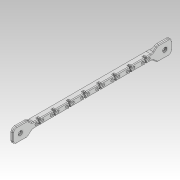
# Autodesk Inventor part: DoubleSolenoidBracket
Saved by Autodesk Inventor 2020 (Build 240168000, 168)
## iProperties
Created: 2021-09-21
Part Number: DoubleSolenoidBracket
Material: Generic
Document SubType Name: Modeling
Designer: DDeGo
Density: 1 g/cm^3
Appearance: Default
Author: DDeGo
Autodesk Inventor part; units mm, degrees
ref_plane "YZ Plane" through (0, 0, 0) normal (1, 0, 0) x (0, 1, 0)
ref_plane "XZ Plane" through (0, 0, 0) normal (0, 1, 0) x (-1, 0, 0)
sketch "Sketch1" plane through (0, 0, 0) normal (1, 0, 0) x (0, 1, 0)
  line L0 (0, 0) -> (8, 0)
  line L1 (8, 0) -> (8, -166)
  line L2 (8, -166) -> (0, -166)
  line L3 (0, -166) -> (0, 0)
  line L4 (4, 0) -> (4, -5) construction
  line L5 (4, -5) -> (4, -14) construction
  circle A0 centre (4, -5) radius 1.75
  circle A1 centre (4, -14) radius 1.75
  line L6 (2.75, -10.5) -> (2.75, -8.5) construction
  line L7 (5.25, -8.5) -> (5.25, -10.5) construction
  line L8 (8, -10.5) -> (5.25, -10.5) construction
  line L9 (2.75, -10.5) -> (0, -10.5) construction
  line L10 (0, -8.5) -> (2.75, -8.5) construction
  line L11 (5.25, -8.5) -> (8, -8.5) construction
  line L12 (5.25, -9.5) -> (2.75, -9.5) construction
  circle A2 centre (4, -35) radius 1.75
  line L13 (2.75, -31.5) -> (2.75, -29.5) construction
  line L14 (5.25, -29.5) -> (5.25, -31.5) construction
  circle A3 centre (4, -26) radius 1.75
  line L15 (4, -26) -> (4, -35) construction
  circle A4 centre (4, -56) radius 1.75
  line L16 (2.75, -52.5) -> (2.75, -50.5) construction
  line L17 (5.25, -50.5) -> (5.25, -52.5) construction
  circle A5 centre (4, -47) radius 1.75
  line L18 (4, -47) -> (4, -56) construction
  circle A6 centre (4, -77) radius 1.75
  line L19 (2.75, -73.5) -> (2.75, -71.5) construction
  line L20 (5.25, -71.5) -> (5.25, -73.5) construction
  circle A7 centre (4, -68) radius 1.75
  line L21 (4, -68) -> (4, -77) construction
  circle A8 centre (4, -98) radius 1.75
  line L22 (2.75, -94.5) -> (2.75, -92.5) construction
  line L23 (5.25, -92.5) -> (5.25, -94.5) construction
  circle A9 centre (4, -89) radius 1.75
  line L24 (4, -89) -> (4, -98) construction
  circle A10 centre (4, -119) radius 1.75
  line L25 (2.75, -115.5) -> (2.75, -113.5) construction
  line L26 (5.25, -113.5) -> (5.25, -115.5) construction
  circle A11 centre (4, -110) radius 1.75
  line L27 (4, -110) -> (4, -119) construction
  circle A12 centre (4, -140) radius 1.75
  line L28 (2.75, -136.5) -> (2.75, -134.5) construction
  line L29 (5.25, -134.5) -> (5.25, -136.5) construction
  circle A13 centre (4, -131) radius 1.75
  line L30 (4, -131) -> (4, -140) construction
  circle A14 centre (4, -161) radius 1.75
  line L31 (2.75, -157.5) -> (2.75, -155.5) construction
  line L32 (5.25, -155.5) -> (5.25, -157.5) construction
  circle A15 centre (4, -152) radius 1.75
  line L33 (4, -152) -> (4, -161) construction
  point P0 (4, -9.5)
  point P1 (5.25, -30.5)
  point P2 (2.75, -30.5)
  point P3 (4, -30.5)
  point P4 (5.25, -51.5)
  point P5 (2.75, -51.5)
  point P6 (4, -51.5)
  point P7 (5.25, -72.5)
  point P8 (2.75, -72.5)
  point P9 (4, -72.5)
  point P10 (5.25, -93.5)
  point P11 (2.75, -93.5)
  point P12 (4, -93.5)
  point P13 (5.25, -114.5)
  point P14 (2.75, -114.5)
  point P15 (4, -114.5)
  point P16 (5.25, -135.5)
  point P17 (2.75, -135.5)
  point P18 (4, -135.5)
  point P19 (5.25, -156.5)
  point P20 (2.75, -156.5)
  point P21 (4, -156.5)
  dimension "d0" = 9
  dimension "d1" = 3.5
  dimension "d2" = 5
  dimension "d3" = 2.5
  dimension "d4" = 2
  dimension "d5" = 8
  dimension "d8" = 21
  dimension "d13" = 5
  constraints: 68 end point, 16 centre point, 16 coincident, 10 perpendicular, 5 midpoint, 5 point on line, 3 parallel, 2 collinear, 1 equal radius, 1 horizontal, 1 vertical, 111 other
  measures "d0" distance of L4.end L5.end
  measures "d1" diameter of A0
  measures "d2" distance of L4.start L4.end
  measures "d3" distance between parallel lines of L6 L7
  measures "d4" distance of L7.start L7.end
  measures "d5" distance between parallel lines of L3 L1
  measures "d8" distance of A1.centre A2.centre
  measures "d13" distance from line of A14.centre L2
extrude "Extrusion1" add sketch "Sketch1" along normal blind 7
sketch "Sketch2" plane through (7, 0, 0) normal (1, 0, 0) x (0, 0, -1)
  circle A0 centre (5, 4) radius 1.75 construction
  circle A1 centre (14, 4) radius 1.75 construction
  line L0 (5, 4) -> (14, 4) construction
  line L1 (8.75, 2.75) -> (10.25, 2.75)
  line L2 (10.25, 2.75) -> (10.25, 5.25) construction
  line L3 (10.25, 5.25) -> (8.75, 5.25)
  line L4 (8.75, 5.25) -> (8.75, 2.75) construction
  line L5 (8.75, 2.75) -> (10.25, 5.25) construction
  line L6 (10.25, 2.75) -> (8.75, 5.25) construction
  line L7 (8.75, 5.25) -> (8.75, 8)
  line L8 (166, 8) -> (0, 8) construction
  line L9 (10.25, 5.25) -> (10.25, 8)
  line L10 (8.75, 8) -> (10.25, 8)
  line L11 (10.25, 2.75) -> (10.25, 0)
  line L12 (0, 0) -> (166, 0) construction
  line L13 (8.75, 2.75) -> (8.75, 0)
  line L14 (10.25, 0) -> (8.75, 0)
  point P0 (9.5, 4)
  dimension "d16" = 2.5
  dimension "d17" = 1.5
  constraints: 26 end point, 6 point on line, 3 midpoint, 3 parallel, 3 perpendicular, 2 horizontal, 1 vertical
  measures "d16" distance between parallel lines of L1 L3
  measures "d17" distance between parallel lines of L4 L2
extrude "Extrusion2" cut sketch "Sketch2" against normal blind 3.5
fillet "Fillet1" radius 1 4 edges at (5.25, 8, -8.75) (5.25, 8, -10.25) (5.25, 0, -8.75) (5.25, 0, -10.25)
fillet "Fillet1" radius 0.5 4 edges at (5.25, 2.75, -8.75) (5.25, 2.75, -10.25) (5.25, 5.25, -8.75) (5.25, 5.25, -10.25)
sketch "Sketch4" plane through (0, 0, 0) normal (-1, 0, 0) x (0, 0, 1)
  circle A0 centre (-5, 4) radius 1.75 projected
  circle A1 centre (-5, 4) radius 3
  circle A2 centre (-14, 4) radius 1.75 projected
  circle A3 centre (-14, 4) radius 3
  point P0 (0, 0)
  dimension "d25" = 6
  constraints: 2 centre point, 2 coincident, 1 equal radius
  measures "d25" diameter of A1
extrude "Extrusion4" cut sketch "Sketch4" against normal blind 3 contours A0 | A1 | A2 | A3
pattern_linear "Rectangular Pattern1" count 8 spacing 21 along (0, 0, -1) of "Extrusion4", "Extrusion2", "Fillet1"
ref_plane "Work Plane1" through (0, 0, -83) normal (0, 0, 1) x (1, 0, 0)
sketch "Sketch5" plane through (7, 0, 0) normal (1, 0, 0) x (0, 0, -1)
  line L0 (0, 0) -> (166, 0) construction
  line L1 (166, 8) -> (0, 8) construction
  line L2 (0, 0) -> (0, 8)
  line L3 (0, 8) -> (-7, 14)
  line L4 (-7, 14) -> (-27, 14)
  line L5 (-27, 14) -> (-27, -6)
  line L6 (-27, -6) -> (-7, -6)
  line L7 (-7, -6) -> (-7, 14) construction
  line L8 (0, 8) -> (0, 0) projected
  line L9 (-7, -6) -> (0, 0)
  line L10 (-7, 4) -> (-27, 4) construction
  circle A0 centre (-17, 4) radius 3
  line L11 (83, -10) -> (83, 18) projected
  dimension "d31" = 6
  dimension "d32" = 20
  dimension "d33" = 100
  dimension "d34" = 20
  constraints: 16 end point, 5 perpendicular, 3 midpoint, 1 centre point, 1 equal length
  measures "d31" diameter of A0
  measures "d32" distance of L4.end L5.end
  measures "d33" distance from line of L11 A0.centre
  measures "d34" distance of L3.end L4.end
extrude "Extrusion5" add sketch "Sketch5" against normal blind 3
mirror "Mirror1" about plane through (0, 0, -83) normal (0, 0, 1) of "Extrusion5"
fillet "Fillet2" radius 5 4 edges at (5.5, 14, 27) (5.5, -6, 27) (5.5, 14, -193) (5.5, -6, -193)
fillet "Fillet2" radius 5 8 edges at (5.5, 14, 7) (5.5, 0, 0) (5.5, 8, 0) (5.5, -6, 7) (5.5, 14, -173) (5.5, 8, -166) (5.5, 0, -166) (5.5, -6, -173)
chamfer "Chamfer1" distance 4 angle 45 2 edges at (4, 4, 0) (4, 4, -166)
fillet "Fillet3" radius 5 2 edges at (4, 4, 3.9999) (4, 4, -169.9999)
fillet "Fillet4" radius 1 152 edges at (7, 0.2929, -10.5429) (7, 0, -20) (7, 0.2929, -29.4571) (7, 1.625, -29.75) (7, 2.6036, -29.8964) (7, 2.75, -30.5) (7, 2.6036, -31.1036) (7, 1.625, -31.25) (7, 0.2929, -31.5429) (7, 0, -41) (7, 0.2929, -50.4571) (7, 1.625, -50.75) (7, 2.6036, -50.8964) (7, 2.75, -51.5) (7, 2.6036, -52.1036) (7, 1.625, -52.25) (7, 0.2929, -52.5429) (7, 0, -62) (7, 0.2929, -71.4571) (7, 1.625, -71.75) (7, 2.6036, -71.8964) (7, 2.75, -72.5) (7, 2.6036, -73.1036) (7, 1.625, -73.25) (7, 0.2929, -73.5429) (7, 0, -83) (7, 0.2929, -92.4571) (7, 1.625, -92.75) (7, 2.6036, -92.8964) (7, 2.75, -93.5) (7, 2.6036, -94.1036) (7, 1.625, -94.25) (7, 0.2929, -94.5429) (7, 0, -104) (7, 0.2929, -113.4571) (7, 1.625, -113.75) (7, 2.6036, -113.8964) (7, 2.75, -114.5) (7, 2.6036, -115.1036) (7, 1.625, -115.25) (7, 0.2929, -115.5429) (7, 0, -125) (7, 0.2929, -134.4571) (7, 1.625, -134.75) (7, 2.6036, -134.8964) (7, 2.75, -135.5) (7, 2.6036, -136.1036) (7, 1.625, -136.25) (7, 0.2929, -136.5429) (7, 0, -146) (7, 0.2929, -155.4571) (7, 1.625, -155.75) (7, 2.6036, -155.8964) (7, 2.75, -156.5) (7, 2.6036, -157.1036) (7, 1.625, -157.25) (7, 0.2929, -157.5429) (7, 0, -161.2002) (7, -0.3106, -165.8851) (7, -3, -169.5) (7, -5.6894, -173.1149) (7, -6, -181.4248) (7, -4.5355, -191.5355) (7, 4, -193) (7, 12.5355, -191.5355) (7, 14, -181.4248) (7, 13.6894, -173.1149) (7, 11, -169.5) (7, 8.3106, -165.8851) (7, 8, -161.2002) (7, 7.7071, -157.5429) (7, 6.375, -157.25) (7, 5.3964, -157.1036) (7, 5.25, -156.5) (7, 5.3964, -155.8964) (7, 6.375, -155.75) (7, 7.7071, -155.4571) (7, 8, -146) (7, 7.7071, -136.5429) (7, 6.375, -136.25) (7, 5.3964, -136.1036) (7, 5.25, -135.5) (7, 5.3964, -134.8964) (7, 6.375, -134.75) (7, 7.7071, -134.4571) (7, 8, -125) (7, 7.7071, -115.5429) (7, 6.375, -115.25) (7, 5.3964, -115.1036) (7, 5.25, -114.5) (7, 5.3964, -113.8964) (7, 6.375, -113.75) (7, 7.7071, -113.4571) (7, 8, -104) (7, 7.7071, -94.5429) (7, 6.375, -94.25) (7, 5.3964, -94.1036) (7, 5.25, -93.5) (7, 5.3964, -92.8964) (7, 6.375, -92.75) (7, 7.7071, -92.4571) (7, 8, -83) (7, 7.7071, -73.5429) (7, 6.375, -73.25) (7, 5.3964, -73.1036) (7, 5.25, -72.5) (7, 5.3964, -71.8964) (7, 6.375, -71.75) (7, 7.7071, -71.4571) (7, 8, -62) (7, 7.7071, -52.5429) (7, 6.375, -52.25) (7, 5.3964, -52.1036) (7, 5.25, -51.5) (7, 5.3964, -50.8964) (7, 6.375, -50.75) (7, 7.7071, -50.4571) (7, 8, -41) (7, 7.7071, -31.5429) (7, 6.375, -31.25) (7, 5.3964, -31.1036) (7, 5.25, -30.5) (7, 5.3964, -29.8964) (7, 6.375, -29.75) (7, 7.7071, -29.4571) (7, 8, -20) (7, 7.7071, -10.5429) (7, 6.375, -10.25) (7, 5.3964, -10.1036) (7, 5.25, -9.5) (7, 5.3964, -8.8964) (7, 6.375, -8.75) (7, 7.7071, -8.4571) (7, 8, -4.7998) (7, 8.3106, -0.1149) (7, 11, 3.5) (7, 13.6894, 7.1149) (7, 14, 15.4248) (7, 12.5355, 25.5355) (7, 4, 27) (7, -4.5355, 25.5355) (7, -6, 15.4248) (7, -5.6894, 7.1149) (7, -3, 3.5) (7, -0.3106, -0.1149) (7, 0, -4.7998) (7, 0.2929, -8.4571) (7, 1.625, -8.75) (7, 2.6036, -8.8964) (7, 2.75, -9.5) (7, 2.6036, -10.1036) (7, 1.625, -10.25)
equation "\"d13\" = d2"
equation "\"d30\" = d8"
body "Solid1"
